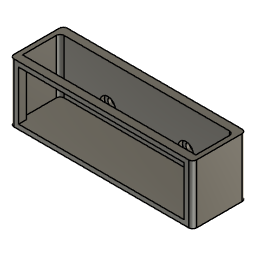
cnc-controller-holder v4 (Autodesk Fusion 360 design; units mm, degrees)
Autodesk Fusion 360 part; units mm, degrees
sketch "controller-mock" plane through (0, 0, 0) normal (0, 1, 0) x (1, 0, 0)
  line L0 (0, 0) -> (106.5, 0)
  line L1 (106.5, 0) -> (106.5, -77.5)
  line L2 (106.5, -77.5) -> (0, -77.5)
  line L3 (0, -77.5) -> (0, 0)
  dimension "d1" = 77.5
  dimension "d2" = 106.5
  constraint horizontal L0
  constraint vertical L1
  constraint horizontal L2
  constraint vertical L3
  constraint coincident L0.start L3.end
  measures "d1" distance of L0.start L2.end
  measures "d2" distance of L0.start L0.end
extrude "Extrude1" add sketch "controller-mock" along normal blind 24 makes body 1
sketch "Sketch2" plane through (0, 0, 0) normal (0, 1, 0) x (1, 0, 0)
  line L0 (106.5, -77.5) -> (0, -77.5)
  line L1 (0, -77.5) -> (0, 0)
  line L2 (0, 0) -> (106.5, 0)
  line L3 (106.5, 0) -> (106.5, -77.5)
  line L4 (53.25, 0) -> (53.25, -77.5) construction
  line L5 (-5, 5) -> (111.5, 5)
  line L6 (111.5, 5) -> (111.5, -82.5)
  line L7 (111.5, -82.5) -> (-5, -82.5)
  line L8 (-5, -82.5) -> (-5, 5)
  dimension "d5" = -5
  constraint midpoint L2 L4.start
  constraint midpoint L0 L4.end
extrude "Extrude2" add sketch "Sketch2" along normal blind 34 separate body contours L0 L1 L2 L3 | L5 L6 L7 L8 makes body 2
sketch "Sketch3" plane through (0, 0, 82.5) normal (0, 0, 1) x (-1, 0, 0)
  line L0 (5, 0) -> (-111.5, 0)
  line L1 (-111.5, 0) -> (-111.5, -34)
  line L2 (-111.5, -34) -> (5, -34)
  line L3 (5, -34) -> (5, 0)
  line L4 (-111.5, -17) -> (5, -17) construction
  line L5 (-111.5, -5) -> (5, -5)
  line L6 (-111.5, -29) -> (5, -29)
  line L7 (-53.25, -17) -> (-53.25, -29) construction
  line L8 (2, -29) -> (2, -5)
  line L9 (-108.5, -29) -> (-108.5, -5)
  dimension "d8" = 5
  dimension "d9" = 3
  constraint midpoint L1 L4.start
  constraint midpoint L3 L4.end
  constraint coincident L1 L5.start
  constraint coincident L3 L5.end
  constraint perpendicular L3 L5
  constraint symmetric L4 L5.start L6.start
  constraint symmetric L4 L5.end L6.end
  constraint midpoint L4 L7.start
  constraint midpoint L6 L7.end
  constraint coincident L6 L8.start
  constraint coincident L5 L8.end
  constraint perpendicular L5 L8
  constraint symmetric L7 L8.start L9.start
  constraint symmetric L7 L8.end L9.end
  measures "d8" distance of L0 L5
  measures "d9" distance of L3 L8
extrude "Extrude3" cut sketch "Sketch3" against normal blind 80 contours L5 L6 L8 L9 bodies 2
extrude "Extrude4" cut 1 faces at (34.8333, 1.6667, 82.5) along direction (0, 0, -1) blind 40 on bodies 2 bodies 2
extrude "Extrude5" cut 1 faces at (34.8333, 1.6667, 42.5) along direction (0, 0, -1) blind 10 on bodies 2 bodies 2
fillet "Fillet1" radius 2.5 2 edges at (-5, 0, 13.75) (111.5, 0, 13.75) on bodies 2
fillet "Fillet3" radius 2.5 2 edges at (-2, 29, 17.5) (108.5, 29, 17.5) on bodies 2
fillet "Fillet4" radius 2.5 2 edges at (111.5, 34, 13.75) (-5, 34, 13.75) on bodies 2
extrude "Extrude6" cut 1 faces at (70.8333, 13, 2.5) along direction (0, 0, -1) blind 4.5 on bodies 2 bodies 2
sketch "Sketch4" plane through (0, 0, 0) normal (0, -1, 0) x (1, 0, 0)
  line L0 (109, -5) -> (109, 32.5)
  line L1 (109, 32.5) -> (-2.5, 32.5)
  line L2 (-2.5, 32.5) -> (-2.5, -5)
  line L3 (-2.5, -5) -> (109, -5)
  line L4 (109, 32.5) -> (-2.5, 32.5)
  line L5 (-2.5, -5) -> (109, -5)
  line L6 (0.5, -2) -> (106, -2)
  line L7 (-2.5, -5) -> (-2.5, 32.5)
  line L8 (109, 32.5) -> (109, -5)
  line L9 (106, -2) -> (106, 32.5)
  line L10 (0.5, -2) -> (0.5, 32.5)
  line L11 (0.5, 29.5) -> (106, 29.5)
  dimension "d26" = 3
  constraint coincident L2.end L3.start
  constraint coincident L1.end L2.start
  constraint coincident L0.end L1.start
  constraint coincident L0.start L3.end
  constraint coincident L6.end L9.start
  constraint coincident L4 L9.end
  constraint perpendicular L4 L9
  constraint coincident L6.start L10.start
  constraint coincident L4 L10.end
  constraint perpendicular L4 L10
  constraint coincident L10 L11.start
  constraint coincident L9 L11.end
  constraint perpendicular L9 L11
  measures "d26" distance of L1 L11
extrude "Extrude7" cut sketch "Sketch4" against normal up to surface (5 mm away) contours L6 L9 L10 L11 bodies 2
sketch "bolt-hole" plane through (0, 29, 0) normal (0, -1, 0) x (1, 0, 0)
  line L0 (106, -2) -> (106, 32.5)
  line L1 (106, 32.5) -> (0.5, 32.5)
  line L2 (0.5, 32.5) -> (0.5, -2)
  line L3 (0.5, -2) -> (106, -2)
  line L4 (53.25, -2) -> (53.25, 32.5) construction
  line L5 (53.25, 15.25) -> (0.5, 15.25) construction
  line L6 (28.375, 23.875) -> (28.375, 7.875) construction
  circle A0 centre (28.375, 7.875) radius 2.75
  circle A1 centre (28.375, 7.875) radius 4.875
  circle A2 centre (78.125, 7.875) radius 4.875
  circle A3 centre (78.125, 7.875) radius 2.75
  dimension "d31" = 5.5
  dimension "d32" = 9.75
  dimension "d37" = 5
  dimension "d38" = 20
  constraint midpoint L1 L4.end
  constraint midpoint L4 L5.start
  constraint coincident L2 L5.end
  constraint perpendicular L2 L5
  constraint coincident L6.end A0.centre
  constraint concentric A0 A1
  constraint midpoint L3 L4.start
  constraint symmetric L4 A0 A3
  constraint symmetric L4 A1 A2
  measures "d31" diameter of A0
  measures "d32" diameter of A1
  measures "d37" distance of L3 A1
  measures "d38" distance of L4 A1
extrude "Extrude8" cut sketch "bolt-hole" against normal up to surface (5 mm away) contours A0 | A3 bodies 2
extrude "Extrude9" cut sketch "bolt-hole" against normal blind 2.75 contours A1 | A2 bodies 2
move_body "Move1" bodies 1 to x (1, 0, 0) y (0, 1, 0) z (0, 0, 1) at (0, 5, 0)
hidden bodies 1
equation "d6 = 24 mm + 10 mm"
named bodies: "controller-mock", "cnc-controller-mount"
